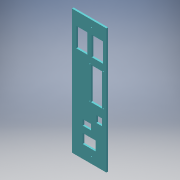
# Autodesk Inventor part: support_arriere
Saved by Autodesk Inventor 2019 (Build 230136000, 136)
## iProperties
Created: 2017-04-21
Part Number: support_arriere
Material: Générique
Document SubType Name: Modeling
Designer: franc
Density: 1 g/cm^3
Appearance: Par défaut
Author: franc
Autodesk Inventor part; units mm, degrees
ref_plane "YZ Plane" through (0, 0, 0) normal (1, 0, 0) x (0, 1, 0)
ref_plane "XZ Plane" through (0, 0, 0) normal (0, 1, 0) x (-1, 0, 0)
ref_plane "XY Plane" through (0, 0, 0) normal (0, 0, 1) x (1, 0, 0)
sketch "Sketch1" plane through (0, 0, 0) normal (0, 1, 0) x (-1, 0, 0)
  line L0 (37.7589, 9.4959) -> (-42.2411, 9.4959)
  line L1 (-42.2411, 9.4959) -> (-42.2411, -280.5041)
  line L2 (-42.2411, -280.5041) -> (37.7589, -280.5041)
  line L3 (27.7589, -20.5041) -> (1.7589, -20.5041)
  line L4 (1.7589, -20.5041) -> (1.7589, -65.5041)
  line L5 (1.7589, -65.5041) -> (27.7589, -65.5041)
  line L6 (27.7589, -65.5041) -> (27.7589, -20.5041)
  line L7 (-8.2411, -20.5041) -> (-34.2411, -20.5041)
  line L8 (-34.2411, -20.5041) -> (-34.2411, -65.5041)
  line L9 (-34.2411, -65.5041) -> (-8.2411, -65.5041)
  line L10 (-8.2411, -65.5041) -> (-8.2411, -20.5041)
  line L11 (-6.2411, -81.8041) -> (-32.2411, -81.8041)
  line L12 (-32.2411, -81.8041) -> (-32.2411, -156.8041)
  line L13 (-32.2411, -156.8041) -> (-6.2411, -156.8041)
  line L14 (-6.2411, -156.8041) -> (-6.2411, -81.8041)
  circle A0 centre (-3.3411, -80.5041) radius 1.5
  circle A1 centre (-34.3411, -80.5041) radius 1.5
  circle A2 centre (-3.3411, -155.5041) radius 1.5
  circle A3 centre (-34.3411, -155.5041) radius 1.5
  line L15 (37.7589, 9.4959) -> (37.7589, -280.5041)
  line L16 (37.7589, -170.5041) -> (37.7589, -280.5041)
  line L17 (12.7589, -228.5041) -> (-17.2411, -228.5041)
  line L18 (-17.2411, -228.5041) -> (-17.2411, -250.5041)
  line L19 (-17.2411, -250.5041) -> (12.7589, -250.5041)
  line L20 (12.7589, -250.5041) -> (12.7589, -228.5041)
  line L21 (12.7589, -200.5041) -> (-6.2411, -200.5041)
  line L22 (-6.2411, -200.5041) -> (-6.2411, -213.5041)
  line L23 (-6.2411, -213.5041) -> (12.7589, -213.5041)
  line L24 (12.7589, -213.5041) -> (12.7589, -200.5041)
  circle A4 centre (-7.2411, -265.5041) radius 1.5
  circle A5 centre (-7.2411, -5.5041) radius 1.5
  point P0 (0, 0)
  dimension "d0" = 290
  dimension "d1" = 80
  dimension "d4" = 45
  dimension "d5" = 26
  dimension "d6" = 30
  dimension "d8" = 45
  dimension "d9" = 26
  dimension "d10" = 30
  dimension "d11" = 10
  dimension "d12" = 75
  dimension "d13" = 26
  dimension "d16" = 1.3
  dimension "d17" = 2.9
  dimension "d18" = 3
  dimension "d20" = 31
  dimension "d22" = 3
  dimension "d23" = 75
  dimension "d24" = 3
  dimension "d25" = 75
  dimension "d26" = 3
  dimension "d27" = 15
  dimension "d28" = 10
  dimension "d32" = 22
  dimension "d33" = 30
  dimension "d34" = 25
  dimension "d35" = 30
  dimension "d36" = 13
  dimension "d37" = 19
  dimension "d38" = 25
  dimension "d39" = 15
  dimension "d40" = 45
  dimension "d41" = 15
  dimension "d42" = 3
  dimension "d43" = 45
  dimension "d44" = 15
  dimension "d45" = 3
  constraints: 50 end point, 11 parallel, 7 perpendicular, 6 centre point, 6 horizontal, 1 point on line, 1 vertical
  measures "d0" distance of L2.end L0.start
  measures "d1" distance of L0.start L0.end
  measures "d4" distance of L5.end L3.start
  measures "d5" distance of L4.end L5.end
  measures "d6" distance between parallel lines of L0 L3
  measures "d8" distance of L9.end L7.start
  measures "d9" distance of L8.end L9.end
  measures "d10" distance between parallel lines of L0 L7
  measures "d11" distance between parallel lines of L10 L4
  measures "d12" distance of L13.end L11.start
  measures "d13" distance of L11.start L11.end
  measures "d16" distance from line of L11 A0.centre
  measures "d17" distance from line of L14 A0.centre
  measures "d18" diameter of A0
  measures "d20" distance of A1.centre A0.centre
  measures "d22" diameter of A1
  measures "d23" distance of A2.centre A0.centre
  measures "d24" diameter of A2
  measures "d25" distance of A3.centre A1.centre
  measures "d26" diameter of A3
  measures "d27" distance from line of L5 A0.centre
  measures "d28" distance between parallel lines of L1 L12
  measures "d32" distance of L19.end L17.start
  measures "d33" distance of L17.start L17.end
  measures "d34" distance between parallel lines of L16 L20
  measures "d35" distance between parallel lines of L2 L19
  measures "d36" distance of L23.end L21.start
  measures "d37" distance of L21.start L21.end
  measures "d38" distance between parallel lines of L16 L24
  measures "d39" distance between parallel lines of L17 L23
  measures "d40" distance from line of L15 A5.centre
  measures "d41" distance from line of L0 A5.centre
  measures "d42" diameter of A5
  measures "d43" distance from line of L16 A4.centre
  measures "d44" distance from line of L2 A4.centre
  measures "d45" diameter of A4
extrude "Extrusion1" add sketch "Sketch1" along normal blind 4
sketch "Esquisse2" plane through (0, 4, 0) normal (0, 1, 0) x (1, 0, 0)
  line L0 (18.8111, 176.8041) -> (32.2411, 176.8041)
  line L1 (32.2411, 176.8041) -> (32.2411, 192.3041)
  line L2 (32.2411, 192.3041) -> (18.8111, 192.3041)
  line L3 (18.8111, 192.3041) -> (18.8111, 176.8041)
  line L4 (42.2411, -9.4959) -> (42.2411, 280.5041) projected
  line L5 (6.2411, 156.8041) -> (32.2411, 156.8041) projected
  point P0 (0, 0)
  dimension "d46" = 15.5
  dimension "d47" = 13.43
  dimension "d48" = 10
  dimension "d49" = 20
  constraints: 8 end point, 2 parallel, 1 horizontal, 1 perpendicular
  measures "d46" distance of L2.end L0.start
  measures "d47" distance of L1.end L2.end
  measures "d48" distance between parallel lines of L4 L1
  measures "d49" distance between parallel lines of L5 L0
extrude "Extrusion2" cut sketch "Esquisse2" against normal through all
body "Solid1"
